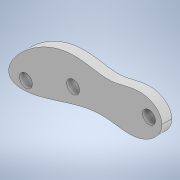
# Autodesk Inventor part: Component33
Saved by Autodesk Inventor 2022 (Build 260153000, 153)
## iProperties
Created: 2022-01-29
Part Number: Component33
Material: Generic
Document SubType Name: Modeling
Designer: Administrator
Density: 1 g/cm^3
Appearance: Default
Title: Component33
Author: Administrator
Autodesk Inventor part; units mm, degrees
ref_plane "YZ Plane" through (0, 0, 0) normal (1, 0, 0) x (0, 1, 0)
ref_plane "XZ Plane" through (0, 0, 0) normal (0, 1, 0) x (-1, 0, 0)
ref_plane "XY Plane" through (0, 0, 0) normal (0, 0, 1) x (1, 0, 0)
sketch "Sketch2" plane through (0, 0, 0) normal (0, 0, 1) x (1, 0, 0)
  circle A0 centre (-27.3479, -10.7746) radius 3.25
  circle A1 centre (34.8208, 4.3138) radius 3.25
  circle A2 centre (-3.4936, -1.5858) radius 3.25
  spline S0 degree 5 poles (41.324, 4.3228) (41.324, 3.6439) (41.1697, 2.2667) (40.4742, 0.1812) (38.6853, -2.4773) (35.4002, -5.2285) (31.535, -7.1363) (27.5171, -8.077) (23.572, -8.1536) (19.6981, -7.6755) (15.7663, -7.045) (11.5874, -6.6671) (6.9873, -6.8581) (1.8924, -7.7332) (-3.6548, -9.206) (-9.5209, -11.0542) (-15.4946, -12.9643) (-21.3038, -14.5846) (-26.6307, -15.5745) (-31.1286, -15.6545) (-34.434, -14.6584) (-36.2298, -12.5463) (-36.3051, -9.4106) (-34.6311, -5.4933) (-31.3878, -1.1726) (-26.8915, 3.1113) (-21.5436, 6.9185) (-15.7714, 9.8751) (-9.9721, 11.7395) (-4.4571, 12.4654) (0.6091, 12.2772) (5.1845, 11.5703) (9.3182, 10.8011) (13.1223, 10.3738) (16.7418, 10.5425) (20.3275, 11.2736) (24.0013, 12.2489) (27.8149, 13.0255) (31.7091, 13.1548) (35.4745, 12.3146) (38.7034, 10.4456) (40.4764, 8.2487) (41.1697, 6.3397) (41.324, 5.0016) (41.324, 4.3228) knots 0 0 0 0 0 0 0.025 0.05 0.075 0.1 0.125 0.15 0.175 0.2 0.225 0.25 0.275 0.3 0.325 0.35 0.375 0.4 0.425 0.45 0.475 0.5 0.525 0.55 0.575 0.6 0.625 0.65 0.675 0.7 0.725 0.75 0.775 0.8 0.825 0.85 0.875 0.9 0.925 0.95 0.975 1 1 1 1 1 1 weights 1 1 1 1 1 1 1 1 1 1 1 1 1 1 1 1 1 1 1 1 1 1 1 1 1 1 1 1 1 1 1 1 1 1 1 1 1 1 1 1 1 1 1 1 1
  point P0 (0, 0)
  dimension "d2" = 6.5
  constraints: 3 centre point, 2 equal radius, 1 other
  measures "d2" diameter of A0
extrude "Extrusion1" add sketch "Sketch2" along normal blind 5
equation "\"d2\" = R"
equation "\"R\" = 6.5"
equation "\"thickness\" = 5"
equation "\"width\" = 6.5"
equation "\"R1\" = 9"
body "Solid2"
